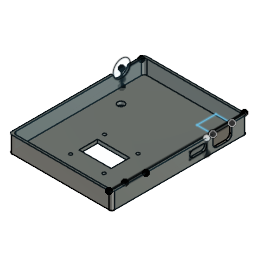
PMSA0031_LID_Casing (Autodesk Fusion 360 design; units mm, degrees)
part number: 2026-03-31-13-21-30-961
Autodesk Fusion 360 part; units mm, degrees
note: some values were not read from the file. Set by a fixed rule: which sketch regions a step uses.
sketch "Sketch1" plane through (0, 0, 0) normal (0, 0, 1) x (1, 0, 0)
  line L0 (36.9, -48.5) -> (-36.9, -48.5)
  line L1 (-36.9, -48.5) -> (-36.9, 48.5)
  line L2 (-36.9, 48.5) -> (36.9, 48.5)
  line L3 (36.9, 48.5) -> (36.9, -48.5)
  line L4 (36.9, -48.5) -> (-36.9, 48.5) construction
  line L5 (-36.9, -48.5) -> (36.9, 48.5) construction
  line L6 (35.35, -46.95) -> (-35.35, -46.95)
  line L7 (-35.35, -46.95) -> (-35.35, 46.95)
  line L8 (-35.35, 46.95) -> (35.35, 46.95)
  line L9 (35.35, 46.95) -> (35.35, -46.95)
  line L10 (35.35, -46.95) -> (-35.35, 46.95) construction
  line L11 (-35.35, -46.95) -> (35.35, 46.95) construction
  line L12 (35.35, -46.95) -> (0, -46.95)
  line L13 (0, -46.95) -> (0, -16.95)
  line L14 (11.5, -10.35) -> (-11.5, -10.35)
  line L15 (-11.5, -10.35) -> (-11.5, -23.55)
  line L16 (-11.5, -23.55) -> (11.5, -23.55)
  line L17 (11.5, -23.55) -> (11.5, -10.35)
  line L18 (11.5, -10.35) -> (-11.5, -23.55) construction
  line L19 (-11.5, -10.35) -> (11.5, -23.55) construction
  line L20 (13.775, -30.9) -> (-13.775, -30.9)
  line L21 (-13.775, -30.9) -> (-13.775, -3)
  line L22 (-13.775, -3) -> (13.775, -3)
  line L23 (13.775, -3) -> (13.775, -30.9)
  line L24 (13.775, -30.9) -> (-13.775, -3) construction
  line L25 (-13.775, -30.9) -> (13.775, -3) construction
  line L26 (13.775, -3) -> (11.975, -3)
  line L27 (-13.775, -3) -> (-11.975, -3)
  line L28 (-13.775, -30.9) -> (-11.975, -30.9)
  line L29 (13.775, -30.9) -> (11.975, -30.9)
  line L30 (-11.975, -30.9) -> (-13.775, -30.9)
  line L31 (-13.775, -30.9) -> (-13.775, -29.1)
  line L32 (-13.775, -29.1) -> (-11.975, -29.1)
  line L33 (-11.975, -29.1) -> (-11.975, -30.9)
  line L34 (11.975, -30.9) -> (13.775, -30.9)
  line L35 (13.775, -30.9) -> (13.775, -29.1)
  line L36 (13.775, -29.1) -> (11.975, -29.1)
  line L37 (11.975, -29.1) -> (11.975, -30.9)
  line L38 (-11.975, -3) -> (-13.775, -3)
  line L39 (-13.775, -3) -> (-13.775, -4.8)
  line L40 (-13.775, -4.8) -> (-11.975, -4.8)
  line L41 (-11.975, -4.8) -> (-11.975, -3)
  line L42 (11.975, -3) -> (13.775, -3)
  line L43 (13.775, -3) -> (13.775, -4.8)
  line L44 (13.775, -4.8) -> (11.975, -4.8)
  line L45 (11.975, -4.8) -> (11.975, -3)
  circle A0 centre (-11.975, -4.8) radius 1.1
  circle A1 centre (11.975, -4.8) radius 1.1
  circle A2 centre (11.975, -29.1) radius 1.1
  circle A3 centre (-11.975, -29.1) radius 1.1
  circle A4 centre (-25, 20) radius 2.45
  point P0 (0, -16.95)
  point P1 (0, -16.95)
  dimension "d1" = 73.8
  dimension "d2" = 97
  dimension "d3" = 70.7
  dimension "d4" = 93.9
  dimension "d48" = 30
  dimension "d49" = 23
  dimension "d50" = 13.2
  dimension "d51" = 27.55
  dimension "d52" = 27.9
  dimension "d53" = 1.8
  dimension "d54" = 1.8
  dimension "d55" = 1.8
  dimension "d56" = 1.8
  dimension "d57" = 1.8
  dimension "d58" = 1.8
  dimension "d59" = 1.8
  dimension "d60" = 1.8
  dimension "d61" = 2.2
  dimension "d62" = 2.2
  dimension "d63" = 2.2
  dimension "d64" = 2.2
  dimension "d67" = 4.9
  constraint horizontal L0
  constraint perpendicular L0 L1
  constraint parallel L0 L2
  constraint parallel L1 L3
  constraint coincident L4 origin
  constraint coincident L5 origin
  constraint horizontal L6
  constraint perpendicular L6 L7
  constraint parallel L6 L8
  constraint parallel L7 L9
  constraint coincident L10 origin
  constraint coincident L11 origin
  constraint midpoint L6 L12.end
  constraint perpendicular L6 L13
  constraint horizontal L14
  constraint perpendicular L14 L15
  constraint parallel L14 L16
  constraint parallel L15 L17
  constraint coincident L18 P1
  constraint coincident L19 P1
  constraint coincident P1 P0
  constraint horizontal L20
  constraint perpendicular L20 L21
  constraint parallel L20 L22
  constraint parallel L21 L23
  constraint coincident L24 P1
  constraint coincident L25 P1
  constraint perpendicular L23 L26
  constraint perpendicular L21 L27
  constraint perpendicular L21 L28
  constraint perpendicular L23 L29
  constraint horizontal L30
  constraint vertical L31
  constraint horizontal L32
  constraint vertical L33
  constraint horizontal L34
  constraint vertical L35
  constraint horizontal L36
  constraint vertical L37
  constraint horizontal L38
  constraint vertical L39
  constraint horizontal L40
  constraint vertical L41
  constraint horizontal L42
  constraint vertical L43
  constraint horizontal L44
  constraint vertical L45
  constraint coincident L40.end L41.start
  constraint coincident L44.end L45.start
  constraint coincident L36.end L37.start
  constraint coincident L32.end L33.start
  measures "d1" distance of L1.end L2.end
  measures "d2" distance of L0.end L1.end
  measures "d3" distance of L7.end L8.end
  measures "d4" distance of L6.end L7.end
  measures "d48" distance of L12.end P1
  measures "d49" distance of L15.end L16.end
  measures "d50" distance of L14.end L15.end
  measures "d51" distance of L21.end L22.end
  measures "d52" distance of L20.end L21.end
  measures "d53" distance of L22.end L26.end
  measures "d54" distance of L21.end L27.end
  measures "d55" distance of L20.end L28.end
  measures "d56" distance of L20.start L29.end
  measures "d57" distance of L28.end L32.end
  measures "d58" distance of L29.end L36.end
  measures "d59" distance of L27.end L40.end
  measures "d60" distance of L26.end L44.end
  measures "d61" diameter of A0
  measures "d62" diameter of A1
  measures "d63" diameter of A2
  measures "d64" diameter of A3
  measures "d67" diameter of A4
extrude "Extrude1" add sketch "Sketch1" along normal blind 2.5 contours L0 L1 L2 L3 | L6 L7 L8 L9 L12 | L14 L15 L16 L17 | L20 L23 L29 L34 L35 L36 L37 A2 | L20 L21 L22 L23 L32 L33 L36 L37 L40 L41 L44 L45 A0 A1 A2 A3 | L36 L37 A2 | L36 L37 A2 | L22 L23 L26 L42 L43 L44 L45 A1 | L20 L21 L28 L30 L31 L32 L33 A3 | L44 L45 A1 | L44 L45 A1 | L32 L33 A3 | L32 L33 A3 | L21 L22 L27 L38 L39 L40 L41 A0 | L40 L41 A0 | L40 L41 A0 | A4
extrude "Extrude2" add sketch "Sketch1" along normal blind 12.7 contours L0 L1 L2 L3
fillet "Fillet1" radius 2 8 edges at (-35.35, 46.95, 7.6) (35.35, 46.95, 7.6) (35.35, -46.95, 7.6) (-35.35, -46.95, 7.6) (-36.9, -48.5, 6.35) (36.9, -48.5, 6.35) (36.9, 48.5, 6.35) (-36.9, 48.5, 6.35)
fillet "Fillet2" radius 1 8 edges at (-36.3142, -47.9142, 0) (0, -48.5, 0) (36.3142, -47.9142, 0) (36.9, 0, 0) (36.3142, 47.9142, 0) (0, 48.5, 0) (-36.3142, 47.9142, 0) (-36.9, 0, 0)
sketch "Sketch2" plane through (0, 0, 12.7) normal (0, 0, 1) x (-1, 0, 0)
  line L0 (33.35, -46.95) -> (-33.35, -46.95)
  arc A0 (-35.35, -44.95) -> (-33.35, -46.95) centre (-33.35, -44.95) ccw
  line L1 (-35.35, -44.95) -> (-35.35, 44.95)
  arc A1 (-33.35, 46.95) -> (-35.35, 44.95) centre (-33.35, 44.95) ccw
  line L2 (-33.35, 46.95) -> (33.35, 46.95)
  arc A2 (35.35, 44.95) -> (33.35, 46.95) centre (33.35, 44.95) ccw
  line L3 (35.35, 44.95) -> (35.35, -44.95)
  arc A3 (33.35, -46.95) -> (35.35, -44.95) centre (33.35, -44.95) ccw
  arc A4 (34.9, -48.5) -> (36.9, -46.5) centre (34.9, -46.5) ccw
  line L4 (36.9, -46.5) -> (36.9, 46.5)
  arc A5 (36.9, 46.5) -> (34.9, 48.5) centre (34.9, 46.5) ccw
  line L5 (34.9, 48.5) -> (-34.9, 48.5)
  arc A6 (-34.9, 48.5) -> (-36.9, 46.5) centre (-34.9, 46.5) ccw
  line L6 (-36.9, 46.5) -> (-36.9, -46.5)
  arc A7 (-36.9, -46.5) -> (-34.9, -48.5) centre (-34.9, -46.5) ccw
  line L7 (-34.9, -48.5) -> (34.9, -48.5)
  line L8 (-34.9, 48.5) -> (-34.9, 37.6)
  line L9 (-34.9, 37.6) -> (-35.35, 37.6)
  line L10 (-35.35, 37.6) -> (-36.9, 37.6)
  line L11 (-36.9, 37.6) -> (-36.9, 24.096)
  line L12 (-36.9, 24.096) -> (-35.35, 24.096)
  line L13 (-35.35, 24.096) -> (-35.35, 37.6)
  line L14 (-34.9, 48.5) -> (-34.9, -48.5)
  line L15 (-34.9, -48.5) -> (-34.9, -37.6)
  line L16 (-34.9, -37.6) -> (-34.9, -24.096)
  line L17 (-34.9, -24.096) -> (-36.4, -24.096)
  line L18 (-36.9, -23.896) -> (-25.5, -23.896)
  line L19 (-25.5, -23.896) -> (-25.5, -37.4)
  line L20 (-25.5, -37.4) -> (-36.9, -37.4)
  line L21 (-36.9, -37.4) -> (-36.9, -23.896)
  line L22 (-36.9, -23.896) -> (-36.9, -19.396)
  line L23 (-34.9, -48.5) -> (-34.9, -37.6)
  line L24 (-34.9, -37.6) -> (-36.9, -37.5994)
  dimension "d13" = 10.9
  dimension "d14" = 13.504
  dimension "d19" = 10.9
  dimension "d20" = 13.504
  dimension "d21" = 1.5
  dimension "d22" = 13.504
  dimension "d31" = 4.5
  dimension "d47" = 10.9
  constraint coincident L5.end A6.start
  constraint perpendicular L5 L8
  constraint coincident L1 L9.end
  constraint perpendicular L1 L9
  constraint horizontal L10
  constraint vertical L11
  constraint horizontal L12
  constraint vertical L13
  constraint coincident L6 L11.end
  constraint coincident A7.end L7.start
  constraint perpendicular L7 L15
  constraint parallel L14 L16
  constraint perpendicular L14 L17
  constraint horizontal L18
  constraint vertical L19
  constraint horizontal L20
  constraint vertical L21
  constraint coincident L6 L18.start
  constraint perpendicular L18 L22
  constraint parallel L16 L23
  constraint coincident L6 L24.end
  measures "d13" distance of L5.end L8.end
  measures "d14" distance of L9.end L12.end
  measures "d19" distance of A7.end L15.end
  measures "d20" distance of L15.end L16.end
  measures "d21" distance of L16.end L17.end
  measures "d22" distance of L18.start L20.end
  measures "d31" distance of L18.start L22.end
  measures "d47" distance of A7.end L15.end
extrude "Extrude5" cut sketch "Sketch2" against normal blind 9.5 contours L1 L14 L16 L17 L20 | L1 L6 L18 L20 L21
fillet "Fillet5" radius 3 2 edges at (36.125, 23.896, 3.2) (36.125, 37.4, 3.2)
sketch "Sketch3" plane through (36.9, 0, 0) normal (1, 0, 0) x (0, 1, 0)
  line L0 (37.4, 12.7) -> (37.4, 6.2)
  arc A0 (34.4, 3.2) -> (37.4, 6.2) centre (34.4, 6.2) ccw
  line L1 (34.4, 3.2) -> (26.896, 3.2)
  arc A1 (23.896, 6.2) -> (26.896, 3.2) centre (26.896, 6.2) ccw
  line L2 (23.896, 6.2) -> (23.896, 12.7)
  line L3 (23.896, 12.7) -> (-46.5, 12.7)
  line L4 (-46.5, 12.7) -> (-46.5, 1)
  line L5 (-46.5, 1) -> (46.5, 1)
  line L6 (46.5, 1) -> (46.5, 12.7)
  line L7 (46.5, 12.7) -> (37.4, 12.7)
  line L8 (23.896, 12.7) -> (19.396, 12.7)
  line L9 (19.396, 12.7) -> (19.396, 2.68)
  line L10 (19.396, 12.7) -> (19.396, 10.19)
  line L11 (19.396, 10.19) -> (7.307, 10.19)
  line L12 (7.307, 10.19) -> (7.307, 5.19)
  line L13 (7.307, 5.19) -> (19.396, 5.19)
  line L14 (19.396, 5.19) -> (19.396, 10.19)
  dimension "d32" = 4.5
  dimension "d33" = 10.02
  dimension "d34" = 2.51
  dimension "d35" = 12.089
  dimension "d36" = 5
  constraint coincident L2.end L3.start
  constraint perpendicular L2 L8
  constraint perpendicular L3 L9
  constraint perpendicular L3 L10
  constraint horizontal L11
  constraint vertical L12
  constraint horizontal L13
  constraint vertical L14
  measures "d32" distance of L2.end L8.end
  measures "d33" distance of L8.end L9.end
  measures "d34" distance of L8.end L10.end
  measures "d35" distance of L10.end L11.end
  measures "d36" distance of L10.end L13.end
extrude "Extrude6" cut sketch "Sketch3" against normal blind 2 contours L9 L11 L12 L13 L14
fillet "Fillet6" radius 2.5 4 edges at (36.125, 7.307, 10.19) (36.125, 19.396, 10.19) (36.125, 19.396, 5.19) (36.125, 7.307, 5.19)
sketch "Sketch4" plane through (-35.35, 0, 0) normal (1, 0, 0) x (0, 1, 0)
  line L0 (-44.95, 12.7) -> (-44.95, 2.5)
  line L1 (-44.95, 2.5) -> (44.95, 2.5)
  line L2 (44.95, 2.5) -> (44.95, 12.7)
  line L3 (44.95, 12.7) -> (-44.95, 12.7)
  line L4 (44.95, 12.7) -> (30.837, 12.7)
  line L5 (30.837, 12.7) -> (30.837, 7.306)
  line L6 (30.837, 12.7) -> (30.837, 2.5)
  line L7 (30.837, 2.5) -> (30.837, 13.991)
  circle A0 centre (30.837, 13.991) radius 6.1
  line L8 (36.7988, 12.7) -> (44.95, 12.7)
  dimension "d41" = 14.113
  dimension "d42" = 5.394
  dimension "d43" = 11.491
  dimension "d44" = 12.2
  constraint coincident L2.end L3.start
  constraint perpendicular L2 L4
  constraint perpendicular L3 L5
  constraint coincident L1 L6.end
  constraint perpendicular L1 L6
  constraint perpendicular L4 L7
  constraint coincident L7.end A0.centre
  constraint coincident L4 L8.start
  constraint coincident A0 L8.start
  measures "d41" distance of L2.end L4.end
  measures "d42" distance of L4.end L5.end
  measures "d43" distance of L6.end L7.end
  measures "d44" diameter of A0
extrude "Extrude7" cut sketch "Sketch4" against normal blind 2 contours L3 L5 L6 L7 A0 | L3 L4 L5 L6 L7 A0
extrude "Extrude8" cut sketch "Sketch1" along normal blind 4 contours L14 L15 L16 L17 | L36 L37 A2 | L36 L37 A2 | L44 L45 A1 | L44 L45 A1 | L32 L33 A3 | L32 L33 A3 | L40 L41 A0 | L40 L41 A0
extrude "Extrude9" cut sketch "Sketch1" along normal blind 5 contours A4
